Autodesk Inventor part; units mm, degrees
(part 2 of 2)
sketch "Sketch7" plane through (62.8428, -38.9521, 0) normal (0.622646, -0.7825036, 0) x (0.7825036, 0.622646, 0)
  line L0 (-2.8351, 13.1572) -> (-1.4062, 13.1572) projected
  line L1 (-1.4062, 13.1572) -> (-1.4062, 0) projected
  line L2 (-1.4062, 0) -> (0, 0) projected
  line L3 (0, 0) -> (0, 43.0784) projected
  line L4 (-3.175, 43.0784) -> (-1.4062, 43.0784) projected
  line L5 (-1.4062, 43.0784) -> (-1.4062, 29.9212) projected
  line L6 (-1.4062, 29.9212) -> (-2.8351, 29.9212) projected
  line L7 (-2.8351, 29.9212) -> (-2.8351, 13.1572) projected
  line L8 (181.0207, 43.0784) -> (181.0207, 0) projected
  line L9 (0, 43.0784) -> (181.0207, 43.0784) projected
  line L10 (0, 0) -> (0, 43.0784) projected
  line L11 (0, 0) -> (181.0207, 0) projected
  line L12 (184.5965, 43.0784) -> (187.2357, 43.0784) projected
  line L13 (187.2357, 43.0784) -> (187.2357, 0) projected
  line L14 (187.2357, 0) -> (184.5965, 0) projected
  line L15 (184.5965, 0) -> (184.5965, 13.1572) projected
  line L16 (184.5965, 13.1572) -> (187.7715, 13.1572) projected
  line L17 (187.7715, 13.1572) -> (187.7715, 29.9212) projected
  line L18 (187.7715, 29.9212) -> (184.5965, 29.9212) projected
  line L19 (184.5965, 29.9212) -> (184.5965, 43.0784) projected
  line L20 (187.7715, 0) -> (184.5965, 0) projected
  line L21 (-3.175, 43.0784) -> (-3.175, 43.0784) projected
  line L22 (187.7715, 0) -> (-3.175, 0)
  line L23 (-3.175, 0) -> (-3.175, 43.0784)
  line L24 (-3.175, 43.0784) -> (187.7715, 43.0784)
  line L25 (187.7715, 43.0784) -> (187.7715, 0)
  point P0 (-24.9214, 0)
  constraints: 8 end point, 2 parallel, 1 horizontal, 1 perpendicular
ref_plane "Work Plane6" through (58.3703, -38.4305, 0) normal (0.7860048, 0.6182204, 0) x (-0.6182204, 0.7860048, 0)
body "Solid1"
